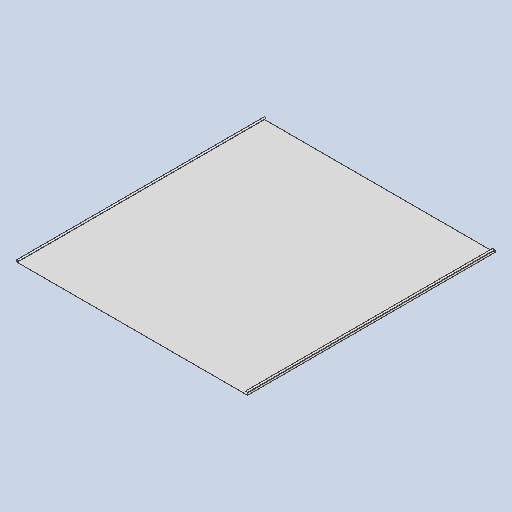
# Autodesk Inventor part: MSC 803 SHEET GILLS
Saved by Autodesk Inventor 2025 (Build 290162010, 162A)
## iProperties
Created: 2024-06-15
Part Number: MSC 803 SHEET GILLS
Material: Stainless Steel
Document SubType Name: Sheet Metal
Designer: pokla
Stock Number: МОО 803 лист жабра
Mass: 3730.66 g
Surface Area: 18672.6 cm^2
Volume: 466.332 cm^3
Density: 8 g/cm^3
Flat Pattern Width: 95.1524 cm
Flat Pattern Length: 98 cm
Flat Pattern Area: 9324.93 cm^2
Sheet Metal Rule: Default_mm
Sheet Metal Width: 951,524 mm
Sheet Metal Length: 980,000 mm
Sheet Metal Area: 932493,416 mm^2
Appearance: Default
Author: pokla
Autodesk Inventor part; units mm, degrees
ref_plane "YZ Plane" through (0, 0, 0) normal (1, 0, 0) x (0, 1, 0)
ref_plane "XZ Plane" through (0, 0, 0) normal (0, 1, 0) x (-1, 0, 0)
ref_plane "XY Plane" through (0, 0, 0) normal (0, 0, 1) x (1, 0, 0)
sketch "Sketch6" plane through (0, 0, 0) normal (0, 1, 0) x (-1, 0, 0)
  line L0 (457.5, -490) -> (-457.5, -490)
  line L1 (-457.5, -490) -> (-457.5, 490)
  line L2 (-457.5, 490) -> (457.5, 490)
  line L3 (457.5, 490) -> (457.5, -490)
  line L4 (457.5, -490) -> (-457.5, 490) construction
  line L5 (-457.5, -490) -> (457.5, 490) construction
  point P0 (0, 0)
  dimension "d52" = 915
  dimension "d53" = 980
  measures "d52" distance of L1.end L2.end
  measures "d53" distance of L0.end L1.end
extrude "Plate2" add sketch "Sketch6" along normal blind 0.5
sketch "Sketch10" plane through (-457, 0, 490) normal (-1, 0, 0) x (0, -1, 0)
  line L0 (0, -980) -> (0, 0)
  line L1 (0, 0) -> (-10, 0)
  line L2 (-10, 0) -> (-10, -980)
  line L3 (-10, -980) -> (0, -980)
  constraints: 6 end point, 1 horizontal, 1 perpendicular, 1 vertical
edge flange "Flange1" height 10 angle 90 thickness 0.5 bend radius 0.5 thickness toward (-1, 0, 0) relief tear relief width 0.5 relief depth 0.25 corner gap 0.5 corner form 0 edges at (-457.5, 0.5, 0) (457.5, 0.5, 0) wall of the first edge with corners at (-457, 0, -490) (-457, 0, 490) (-457, 10, 490) (-457, 10, -490)
bend "Bend2"
corner "Corner2"
sketch "Sketch11" plane through (457.5, 9.5, -490) normal (0, 1, 0) x (-1, 0, 0)
  line L0 (0, 980) -> (0, 0)
  line L1 (0, 0) -> (10, 0)
  line L2 (10, 0) -> (10, 980)
  line L3 (10, 980) -> (0, 980)
  constraints: 6 end point, 1 horizontal, 1 perpendicular, 1 vertical
edge flange "Flange2" height 10 angle 90 thickness 0.5 bend radius 0.5 thickness toward (0, 1, 0) relief tear relief width 0.5 relief depth 0.25 corner gap 0.5 corner form 0 edges at (457, 10, 0) (-457, 10, 0) wall of the first edge with corners at (457.5, 9.5, 490) (457.5, 9.5, -490) (447.5, 9.5, -490) (447.5, 9.5, 490)
bend "Bend3"
corner "Corner3"
sketch "Sketch12" plane through (0, 0, 0) normal (0, -1, 0) x (1, 0, 0)
  line L0 (457.5, -490) -> (457.5, 490) projected
  line L1 (457.5, 490) -> (457.5, -490) projected
  line L2 (-457.5, -490) -> (-457.5, 490) projected
  line L3 (-457.5, 490) -> (-417.5, 490)
  line L4 (-417.5, 490) -> (-417.5, 390)
  line L5 (-417.5, 390) -> (-457.5, 390)
  line L6 (-457.5, 390) -> (-457.5, 490)
  line L7 (457.5, 490) -> (417.5, 490)
  line L8 (417.5, 490) -> (417.5, 390)
  line L9 (417.5, 390) -> (457.5, 390)
  line L10 (457.5, 390) -> (457.5, 490)
  point P0 (0, 0)
  point P1 (-457.5, 30.3845)
  point P2 (457.5, 390)
  point P3 (457.5, 490)
  dimension "d96" = 100
  dimension "d97" = 40
  dimension "d98" = 100
  dimension "d99" = 40
  constraints: 16 end point, 4 parallel, 2 horizontal, 2 perpendicular, 1 point on line
  measures "d96" distance between parallel lines of L3 L5
  measures "d97" distance of L4.end L5.end
  measures "d98" distance between parallel lines of L7 L9
  measures "d99" distance of L8.end L9.end
extrude "Extrusion3" [suppressed]
fillet "Corner Round1" radius 4 4 edges at (447.5, 9.75, 490) (-447.5, 9.75, 490) (447.5, 9.75, -490) (-447.5, 9.75, -490)
equation "\"d52\" = ЖАБРЫ_базовая_ширина"
equation "\"d53\" = ЖАБРЫ_базовая_длина_кор_лист"
equation "\"d98\" = d96"
equation "\"d99\" = d97"
equation "\"d54\" = Thickness"
equation "\"d74\" = BendReliefWidth"
equation "\"d75\" = BendReliefDepth"
equation "\"d76\" = MinimumRemnant"
equation "\"d77\" = TransitionRadius"
equation "\"d80\" = BendRadius"
equation "\"d81\" = CornerReliefSize"
equation "\"d82\" = GapSize"
equation "\"d83\" = JacobiRadiusSize"
equation "\"d84\" = BendReliefWidth"
equation "\"d85\" = BendReliefDepth"
equation "\"d86\" = MinimumRemnant"
equation "\"d87\" = TransitionRadius"
equation "\"d90\" = BendRadius"
equation "\"d91\" = CornerReliefSize"
equation "\"d92\" = GapSize"
equation "\"d93\" = JacobiRadiusSize"
equation "\"BendRadius\" = Thickness"
equation "\"BendReliefWidth\" = Thickness"
equation "\"BendReliefDepth\" = 0.5 * Thickness"
equation "\"CornerReliefSize\" = 4 * Thickness"
equation "\"MinimumRemnant\" = 2 * Thickness"
equation "\"TransitionRadius\" = BendRadius"
equation "\"JacobiRadiusSize\" = BendRadius"
equation "\"GapSize\" = Thickness"
equation "\"ЖАБРЫ_базовая_ширина\" = 915"
equation "\"ЖАБРЫ_базовая_длина_кор_лист\" = 980"
equation "\"Thickness\" = 0.5"
body "Solid2"
